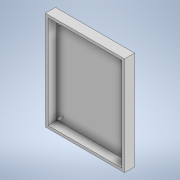
# Autodesk Inventor part: Box
Saved by Autodesk Inventor 2021 (Build 250183000, 183)
## iProperties
Created: 2020-11-03
Part Number: Box
Material: Generic
Document SubType Name: Modeling
Designer: faiya
Density: 1 g/cm^3
Appearance: Default
Author: faiya
Autodesk Inventor part; units mm, degrees
ref_plane "YZ Plane" through (0, 0, 0) normal (1, 0, 0) x (0, 1, 0)
ref_plane "XZ Plane" through (0, 0, 0) normal (0, 1, 0) x (-1, 0, 0)
ref_plane "XY Plane" through (0, 0, 0) normal (0, 0, 1) x (1, 0, 0)
sketch "Sketch1" plane through (0, 0, 0) normal (0, 0, 1) x (1, 0, 0)
  line L0 (0, 0) -> (0, 70.6882)
  line L1 (0, 70.6882) -> (-55.9816, 70.6882)
  line L2 (-55.9816, 70.6882) -> (-55.9816, 0)
  line L3 (-55.9816, 0) -> (0, 0)
  line L4 (-58.0136, 72.7202) -> (2.032, 72.7202)
  line L5 (2.032, 72.7202) -> (2.032, -2.032)
  line L6 (2.032, -2.032) -> (-58.0136, -2.032)
  line L7 (-58.0136, -2.032) -> (-58.0136, 72.7202)
  dimension "d0" = 70.6882
  dimension "d1" = 55.9816
  dimension "d2" = 70.6882
  dimension "d3" = 2.032
  constraints: 16 end point, 4 perpendicular, 1 vertical, 3 other
  measures "d0" distance of L0.start L0.end
  measures "d1" distance of L0.end L1.end
  measures "d2" distance of L1.end L2.end
  measures "d3" distance between parallel lines of L1 L4
extrude "Extrusion1" add sketch "Sketch1" along normal mid plane 7.62
sketch "Sketch2" plane through (-55.9816, 0, 3.81) normal (1, 0, 0) x (0, 0, -1)
  line L0 (7.62, 72.7202) -> (0, 72.7202) projected
  line L1 (7.62, 72.7202) -> (6.858, 72.7202)
  line L2 (7.62, 70.6882) -> (0, 70.6882) projected
  line L3 (7.62, 70.6882) -> (6.7695, 70.6882)
  line L4 (6.7695, 70.6882) -> (6.7695, 0)
  line L5 (7.62, 0) -> (0, 0) projected
  line L6 (6.7695, 0) -> (7.62, 0)
  line L7 (7.62, 70.6882) -> (7.62, 0) projected
  line L8 (7.62, 0) -> (7.62, 70.6882)
  line L9 (7.62, 0) -> (7.62, 70.6882) projected
  line L10 (7.62, 70.6882) -> (6.8499, 70.6882)
  line L11 (0, 0) -> (7.62, 0) projected
  line L12 (6.7695, 0) -> (7.62, 0)
  line L13 (7.62, 0) -> (7.62, 70.6882)
  line L14 (6.6596, 0) -> (7.62, 0)
  line L15 (7.62, 72.7202) -> (7.62, -2.032) projected
  point P0 (3.81, 0)
  dimension "d6" = 0.762
  dimension "d7" = 70.6882
  constraints: 18 end point, 4 point on line, 3 perpendicular, 1 collinear
  measures "d6" distance of L0.start L1.end
  measures "d7" distance of L3.end L4.end
extrude "Extrusion2" add sketch "Sketch2" along normal blind 55.9816
sketch "Sketch3" plane through (-55.9816, 0, -2.9595) normal (0, 0, 1) x (1, 0, 0)
  line L0 (55.9816, 0) -> (0, 0) projected
  line L1 (55.9816, 70.6882) -> (55.9816, 0) projected
  circle A0 centre (51.9176, 4.064) radius 0.635
  line L2 (0, 0) -> (0, 70.6882) projected
  line L3 (0, 0) -> (0, 4.064)
  circle A1 centre (4.064, 4.064) radius 0.635
  line L4 (0, 70.6882) -> (55.9816, 70.6882) projected
  circle A2 centre (4.064, 66.6242) radius 0.635
  line L5 (55.9816, 70.6882) -> (55.9816, 66.6242)
  circle A3 centre (51.9176, 66.6242) radius 0.635
  dimension "d12" = 1.27
  dimension "d15" = 1.27
  dimension "d18" = 1.27
  dimension "d21" = 1.27
  constraints: 4 centre point, 4 end point, 1 point on line
  measures "d12" diameter of A0
  measures "d15" diameter of A1
  measures "d18" diameter of A2
  measures "d21" diameter of A3
extrude "Extrusion3" add sketch "Sketch3" along normal blind 3.048 contours A0 | A1 | A2 | A3
body "Solid1"
